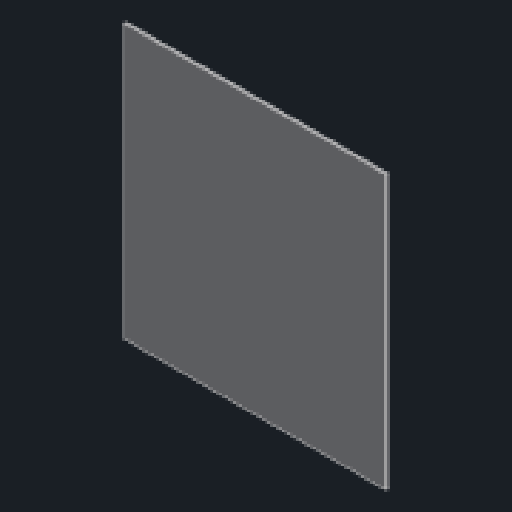
# Autodesk Inventor part: ChestTopPanel
Saved by Autodesk Inventor 2025.2 (Build 292293000, 293)
## iProperties
Created: 2025-10-05
Part Number: ChestTopPanel
Material: Generic
Document SubType Name: Sheet Metal
Designer: valer
Density: 1 g/cm^3
Sheet Metal Rule: Default
Appearance: Default
Author: valer
Autodesk Inventor part; units mm, degrees
ref_plane "YZ Plane" through (0, 0, 0) normal (1, 0, 0) x (0, 1, 0)
ref_plane "XZ Plane" through (0, 0, 0) normal (0, 1, 0) x (-1, 0, 0)
ref_plane "XY Plane" through (0, 0, 0) normal (0, 0, 1) x (1, 0, 0)
sketch "Base" plane through (0, 0, 0) normal (0, 0, 1) x (1, 0, 0)
  line L0 (370.5814, -184.5855) -> (20.5814, -184.5855)
  line L1 (20.5814, -184.5855) -> (20.5814, 180.4145)
  line L2 (20.5814, 180.4145) -> (370.5814, 180.4145)
  line L3 (370.5814, 180.4145) -> (370.5814, -184.5855)
  point P0 (0, 0)
  dimension "d1" = 365
  dimension "d3" = 350
  measures "d1" distance of L2.end L0.start
  measures "d3" distance of L0.start L0.end
extrude "Plate1" add sketch "Base" along normal blind 3.048
chamfer "BaseChamfersFeature" distance 25 angle 45 4 edges at (20.5814, 180.4145, 1.524) (370.5814, 180.4145, 1.524) (370.5814, -184.5855, 1.524) (20.5814, -184.5855, 1.524)
fillet "BaseFilletsFeature" radius 8 8 edges at (20.5814, 155.4145, 1.524) (45.5814, 180.4145, 1.524) (20.5814, -159.5855, 1.524) (45.5814, -184.5855, 1.524) (345.5814, 180.4145, 1.524) (370.5814, 155.4145, 1.524) (370.5814, -159.5855, 1.524) (345.5814, -184.5855, 1.524)
equation "\"d4\" = Thickness"
equation "\"BendRadius\" = Thickness"
equation "\"BendReliefWidth\" = Thickness"
equation "\"BendReliefDepth\" = 0.5 * Thickness"
equation "\"CornerReliefSize\" = 4 * Thickness"
equation "\"MinimumRemnant\" = 2 * Thickness"
equation "\"TransitionRadius\" = BendRadius"
equation "\"JacobiRadiusSize\" = BendRadius"
equation "\"GapSize\" = Thickness"
equation "\"Thickness\" = 3.048"
body "Solid1"
